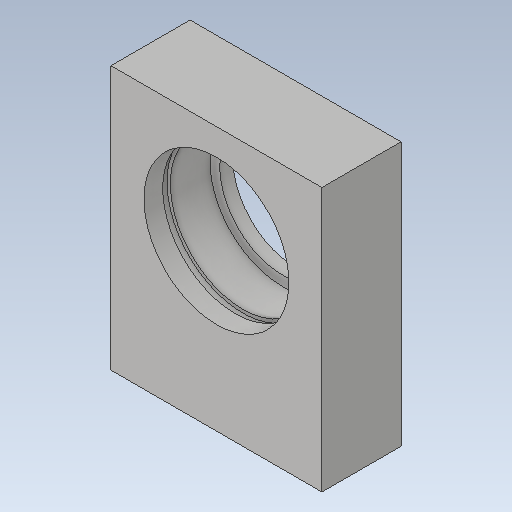
# Autodesk Inventor part: BGBFS6900DD-25-_h
Saved by Autodesk Inventor 2020.2 (Build 242310000, 310)
## iProperties
Created: 2022-11-04
Part Number: BGBFS6900DD-25-_h
Material: Generic
Catalog Web Link: www.cadenas.de
Description: BGBFB, BGBF, BGBFA, BGBFSA, BGBFS_housing-Bearings with Housings - Bottom Mount - h Configurable
Vendor: MISUMI
Document SubType Name: Modeling
Designer: psAdmin
Manufacturer: MISUMI
Mass: 10.6692 g
Surface Area: 48.6357 cm^2
Volume: 10.6692 cm^3
Density: 1 g/cm^3
Appearance: PSOLRGB-175-175-175
Category: PARTsolutions
Company: MISUMI
PSOL_IDENT_0: {$CADENAS_DATA/23d-libs/misumi/metric/12_bearing_holders/bgbfb/bgbfb_housing.prj},245 {VTYP=3D},{NB=
PSOL_IDENT_1: BGBFS6900DD-25-_h},{LINA=BGBFS6900DD-25-},{NN=BGBFB, BGBF, BGBFA, BGBFSA, BGBFS_housing},{DATE=18.09
PSOL_IDENT_2: .2019 08:57:38},{GEOMDATE=09.09.2019 09:39:18},{VERSION=},{LINEID=90},{WBVAR=MATB,MATH,STH,SEAL,HH,A
PSOL_IDENT_3: LT1,ALT2,ALT3},{WBNUMERIC=HH}  {NB=BGBFS6900DD-25-_h},{LINA=BGBFS6900DD-25-},{KT=DUMMY},{PN=BGBFS690
PSOL_IDENT_4: 0DD-25-},{TYPE=BGBFS},{MATB=SS},{MATBALG='S','Steel','SS','Stainless Steel'},{MATH=SUS304},{MATHALG='
PSOL_IDENT_5: 2017AA','2017 Aluminum Alloy','SUS304','304 Stainless Steel'},{STH=-},{STHALG='-','-'},{ARR=304 Stai
PSOL_IDENT_6: nless Steel},{ARR3D=-S},{BN=6900},{SEAL=DD},{SEALALG='ZZ','ZZ(Double Shielded)','VV','VV(Non-Contact
PSOL_IDENT_7: Sealed Rubber Seal)','DD','DD(Contact Sealed Rubber Seal)'},{HH=25},{HHALG=[25:50/1]},{DD=10},{D=22
PSOL_IDENT_8: },{DDHH=19},{B=6},{H=40},{H2=15},{L=32},{L1=20},{T=12},{M=M5},{M3D=5},{PITCH=0.8},{ALT1=},{KKC=0},{A
PSOL_IDENT_9: LT2=},{MM=1.15},{DD2=23},{ALT3=},{ALT1ALG= '', 'Bearings, Retaining Rings Assembled', '-NA'  , 'with
PSOL_IDENT_10: NA (Bearings, Retaining Rings Not Assembled)'},{ALT2ALG= '','w/o KCC (C2 Chamfer)','-KCC','with KCC
PSOL_IDENT_11: (C2 Chamfer)' },{ALT3ALG= '','w/o KKC (C Chamfer)','-KKC','with KKC (C Chamfer)' }
NB: BGBFS6900DD-25-_h
NN: BGBFB, BGBF, BGBFA, BGBFSA, BGBFS_housing
NT: Bearings with Housings - Bottom Mount - h Configurable
NBSYN: $PN._h
LINA: BGBFS6900DD-25-
CATALOG: Misumi
PN: BGBFS6900DD-25-
MATB: Stainless Steel
MATH: 304 Stainless Steel
STH: -
ARR: 304 Stainless Steel
BN: 6900
SEAL: DD(Contact Sealed Rubber Seal)
HH: 25
DD: 10
D: 22
DDHH: 19
B: 6
H: 40
L: 32
L1: 20
T: 12
M: M5
ALT1: Bearings, Retaining Rings Assembled
ALT2: w/o KCC (C2 Chamfer)
ALT3: w/o KKC (C Chamfer)
SUPPLIER: MISUMI
ARTICLENO: BGBFS6900DD-25-_h
BOMINFO: BGBFS6900DD-25-
CREATOR: CADENAS GmbH
Title: BGBFS6900DD-25-
Author: Cadenas PARTsolutions
Comments: Bearings with Housings - Bottom Mount - h Configurable
Autodesk Inventor part; units mm, degrees
sketch "_____1" plane through (0, 0, 0) normal (0, 0, 1) x (1, 0, 0)
  line L0 (-16, 15) -> (-16, -25)
  line L1 (-16, -25) -> (16, -25)
  line L2 (16, -25) -> (16, 15)
  line L3 (16, 15) -> (-16, 15)
  constraints: 8 end point
extrude "Extrusion1" add sketch "_____1" along normal mid plane 12
sketch "Sketch_2" plane through (0, 0, 0) normal (1, 0, 0) x (0, 1, 0)
  line L0 (0, -6) -> (0, 6)
  line L1 (0, 6) -> (11, 6)
  line L2 (11, 6) -> (11, 3.15)
  line L3 (11, 3.15) -> (11.5, 3.15)
  line L4 (11.5, 3.15) -> (11.5, 2)
  line L5 (11.5, 2) -> (11, 2)
  line L6 (11, 2) -> (11, -4)
  line L7 (11, -4) -> (9.5, -4)
  line L8 (9.5, -4) -> (9.5, -6)
  line L9 (9.5, -6) -> (0, -6)
  line L10 (0, -6) -> (0, 6)
  constraints: 22 end point
revolve "Revolution1" cut sketch "Sketch_2" angle 360 about axis through (0, 0, -6) along (0, 0, -1)
sketch "Sketch3" plane through (-16, -25, 6) normal (0, -1, 0) x (1, 0, 0)
  point P0 (6, -6)
hole "Hole1" at (-10, -25, 0) direction (0, 1, 0) diameter 4.134 depth 10 tip angle 120 countersink diameter 5 countersink angle 90 thread size "M5x0.8" class "6H" standard "ISO Metric profile"
pattern_linear "Rectangular Pattern1" count 2 spacing 20 along (1, 0, 0) of "Hole1"
ref_plane "to_bearing_XY" through (0, 0, -4) normal (0, 0, -1) x (1, 0, 0)
ref_plane "to_bearing_YZ" through (0, 0, -4) normal (1, 0, 0) x (0, -1, 0)
ref_plane "to_bearing_ZX" through (0, 0, -4) normal (0, -1, 0) x (0, 0, -1)
ref_plane "to_ring_XY" through (0, 0, 2) normal (0, 0, -1) x (1, 0, 0)
ref_plane "to_ring_YZ" through (0, 0, 2) normal (1, 0, 0) x (0, -1, 0)
ref_plane "to_ring_ZX" through (0, 0, 2) normal (0, -1, 0) x (0, 0, -1)
body "Solid1"
